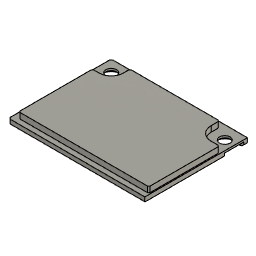
Filament Inlet (Autodesk Fusion 360 archive; units mm, degrees)
design "Inlet Lid"
Autodesk Fusion 360 part; units mm, degrees
sketch "Skizze1" plane through (0, 0, -2) normal (0, 0, 1) x (-1, 0, 0)
  line L0 (-42, -30.1) -> (2.4, -30.1)
  line L1 (2.4, -30.1) -> (2.4, 2.4)
  line L2 (2.4, 2.4) -> (-42, 2.4)
  line L3 (-42, 2.4) -> (-42, -30.1)
  line L4 (0.8, 0.8) -> (-40.4, 0.8)
  line L5 (-40.4, 0.8) -> (-40.4, -28.5)
  line L6 (-40.4, -28.5) -> (0.8, -28.5)
  line L7 (0.8, -28.5) -> (0.8, 0.8)
  dimension "d1" = -1.6
sketch "Skizze2" plane through (0, 0, -2) normal (0, 0, -1) x (1, 0, 0)
  line L0 (42, -30.1) -> (42, 2.4)
  line L1 (42, 2.4) -> (-2.4, 2.4)
  line L2 (-2.4, 2.4) -> (-2.4, -30.1)
  line L3 (-2.4, -30.1) -> (42, -30.1)
  line L4 (-0.6, 0.6) -> (40.2, 0.6)
  line L5 (40.2, 0.6) -> (40.2, -28.3)
  line L6 (40.2, -28.3) -> (-0.6, -28.3)
  line L7 (-0.6, -28.3) -> (-0.6, 0.6)
extrude "Extrusion1" add sketch "Skizze2" along normal blind 1.8 contours L0 L1 L2 L3 | L4 L5 L6 L7
extrude "Extrusion2" add sketch "Skizze1" along normal blind 1.8 contours L4 L5 L6 L7
chamfer "Fase1" distance 0.48 angle 45 6 edges at (19.8, 30.1, -3.8) (-2.4, 13.85, -3.8) (19.8, -2.4, -3.8) (42, 13.85, -3.8) (-2.4, 30.1, -2.9) (-2.4, -2.4, -2.9)
sketch "Skizze3" plane through (0, 0, -3.8) normal (0, 0, -1) x (1, 0, 0)
  line L0 (41.52, 1.92) -> (-1.92, 1.92)
  line L1 (-1.92, 1.92) -> (-1.92, -29.62)
  line L2 (-1.92, -29.62) -> (41.52, -29.62)
  line L3 (41.52, -29.62) -> (41.52, 1.92)
  line L4 (-2.4, 1.92) -> (-2.4, -29.62) construction
  line L5 (-1.92, -30.1) -> (42, -30.1) construction
  circle A0 centre (1.35, -26.35) radius 1.7
  circle A1 centre (1.35, -26.35) radius 3
  circle A2 centre (37.8, -25.9) radius 1.7
  circle A3 centre (37.8, -25.9) radius 3
  line L6 (42, -30.1) -> (42, 2.4)
  dimension "d2" = 3.4
  dimension "d3" = 3.75
  dimension "d4" = 3.75
  dimension "d5" = 6
  dimension "d6" = 3.4
  dimension "d7" = 6
  dimension "d8" = 4.2
  dimension "d9" = 4.2
  constraint concentric A0 A1
  constraint concentric A2 A3
  measures "d2" diameter of A0
  measures "d3" distance of L4 A0.centre
  measures "d4" distance of L5 A0.centre
  measures "d5" diameter of A1
  measures "d6" diameter of A2
  measures "d7" diameter of A3
  measures "d8" distance of A2.centre L6
  measures "d9" distance of L5 A2.centre
extrude "Extrusion3" cut sketch "Skizze3" against normal blind 3.6 contours A0 | A2
chamfer "Fase2" distance 0.4 angle 45 4 edges at (-0.8, 28.5, -1.1) (40.4, -0.8, -1.1) (40.4, 28.5, -1.1) (-0.8, -0.8, -1.1)
extrude "Extrusion4" cut sketch "Skizze3" against normal blind 1.2 contours A1 | A3
sketch "Skizze4" plane through (0, 0, -0.2) normal (0, 0, 1) x (-1, 0, 0)
  circle A0 centre (-37.8, -25.9) radius 1.7
  circle A1 centre (-1.35, -26.35) radius 1.7
  line L0 (0.8, 0.4) -> (0.4, 0.8)
  line L1 (0.4, 0.8) -> (-40, 0.8)
  line L2 (-40, 0.8) -> (-40.4, 0.4)
  line L3 (-40.4, 0.4) -> (-40.4, -28.1)
  line L4 (-40.4, -28.1) -> (-40, -28.5)
  line L5 (-40, -28.5) -> (0.4, -28.5)
  line L6 (0.4, -28.5) -> (0.8, -28.1)
  line L7 (0.8, -28.1) -> (0.8, 0.4)
  circle A2 centre (-1.35, -26.35) radius 3.8
  line L8 (-5.15, -28.5) -> (-5.15, -26.35)
  line L9 (-1.35, -22.55) -> (0.8, -22.55)
  circle A3 centre (-37.8, -25.9) radius 4.3
  line L10 (-33.5, -28.5) -> (-33.5, -25.9)
  line L11 (-40.4, -21.6) -> (-37.8, -21.6)
  dimension "d15" = 7.6
  dimension "d16" = 8.6
  constraint concentric A1 A2
  constraint coincident L5 L8.start
  constraint coincident A2 L8.end
  constraint tangent A2 L8
  constraint coincident A2 L9.start
  constraint coincident L7 L9.end
  constraint tangent A2 L9
  constraint perpendicular L5 L8
  constraint perpendicular L7 L9
  constraint concentric A0 A3
  constraint coincident L5 L10.start
  constraint coincident A3 L10.end
  constraint tangent A3 L10
  constraint coincident L3 L11.start
  constraint coincident A3 L11.end
  constraint tangent A3 L11
  constraint perpendicular L3 L11
  constraint perpendicular L5 L10
  measures "d15" diameter of A2
  measures "d16" diameter of A3
extrude "Extrusion5" cut sketch "Skizze4" against normal blind 1.8 contours L7 A2 L9 | L5 L6 L7 A2 | L5 A2 L8 | L3 A3 L11 | L3 L4 L5 A3 | L3 L4 L5 A3 | L5 A3 L10 picked at (-1.5726, -23.2645)
chamfer "Fase3" distance 0.4 angle 45 4 edges at (40.4, 21.6, -1.1) (33.5, 28.5, -1.1) (5.15, 28.5, -1.1) (-0.8, 22.55, -1.1)
delete_face "Fläche löschen1" 1 faces at (41.84, 8.5933, -3.48)
extrude "Extrusion6" cut 1 faces at (42, 19.1067, -2.6) along direction (-1, 0, 0) blind 1.25
chamfer "Fase5" distance 2.5 angle 45 2 edges at (40.75, 25.3546, -3.2) (40.75, 26.4454, -3.2)
chamfer "Fase6" distance 0.4 angle 45 2 edges at (40.75, 10.4673, -3.8) (40.75, 29.2827, -3.8)
equation "d20 = -2.4 mm + 1.15 mm"
